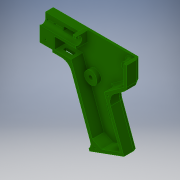
# Autodesk Inventor part: Griff_rechts
Saved by Autodesk Inventor 2019 (Build 230136000, 136)
## iProperties
Created: 2021-03-07
Part Number: Griff_rechts
Material: Generic
Document SubType Name: Modeling
Designer: Lukas
Density: 1 g/cm^3
Appearance: Default
Author: Lukas
Autodesk Inventor part; units mm, degrees
ref_plane "YZ Plane" through (0, 0, 0) normal (1, 0, 0) x (0, 1, 0)
ref_plane "XZ Plane" through (0, 0, 0) normal (0, 1, 0) x (-1, 0, 0)
ref_plane "XY Plane" through (0, 0, 0) normal (0, 0, 1) x (1, 0, 0)
sketch "Sketch1" plane through (0, 0, 0) normal (0, 0, 1) x (1, 0, 0)
  line L0 (-51.5891, 42.2862) -> (-20.8072, -42.2862)
  line L1 (-20.8072, -42.2862) -> (-24.5184, -46.7089)
  line L2 (-24.5184, -46.7089) -> (-23.4923, -49.528)
  line L3 (-23.4923, -49.528) -> (23.4923, -32.427)
  line L4 (27.261, 47.2862) -> (1.261, 28.653)
  line L5 (1.261, 28.653) -> (23.4923, -32.427)
  line L6 (0, -74.8908) -> (0, 102.649) projected
  line L7 (-91.5891, 77.2862) -> (27.261, 77.2862)
  line L8 (27.261, 77.2862) -> (27.261, 47.2862)
  line L9 (-51.5891, 42.2862) -> (-91.5891, 42.2862)
  line L10 (-91.5891, 42.2862) -> (-91.5891, 77.2862)
  point P0 (0, 0)
  point P1 (-36.1981, 0)
  point P2 (0, -40.9775)
  dimension "d1" = 90
  dimension "d2" = 120
  dimension "d3" = 3
  dimension "d5" = 45
  dimension "d6" = 20
  dimension "d7" = 65
  dimension "d8" = 5
  dimension "d10" = 30
  dimension "d30" = 26
  dimension "d31" = 40
  dimension "d32" = 35
  constraints: 21 end point, 5 perpendicular, 2 midpoint, 1 horizontal, 1 horizontal alignment, 1 parallel, 1 vertical alignment
  measures "d1" distance of L0.start L0.end
  measures "d2" angle of L0 L1
  measures "d3" distance of L1.end L2.end
  measures "d5" distance between parallel lines of L5 L0
  measures "d6" angle of L6 L0
  measures "d7" distance of L4.end L3.end
  measures "d8" distance between parallel lines of L2 L0
  measures "d10" distance of L7.end L4.start
  measures "d30" distance from line of L8 L4.end
  measures "d31" distance of L0.start L9.end
  measures "d32" distance of L9.end L7.start
extrude "Extrusion1" add sketch "Sketch1" along normal blind 2.5
sketch "Sketch2" plane through (0, 0, 2.5) normal (0, 0, 1) x (1, 0, 0)
  line L0 (-51.5891, 42.2862) -> (-20.8072, -42.2862) projected
  line L1 (-20.8072, -42.2862) -> (-24.5184, -46.7089) projected
  line L2 (-24.5184, -46.7089) -> (-23.4923, -49.528) projected
  line L3 (-23.4923, -49.528) -> (23.4923, -32.427) projected
  line L4 (23.4923, -32.427) -> (1.261, 28.653) projected
  line L5 (1.261, 28.653) -> (27.261, 47.2862) projected
  line L6 (27.261, 47.2862) -> (27.261, 77.2862) projected
  line L7 (27.261, 77.2862) -> (-91.5891, 77.2862) projected
  circle A0 centre (-32, 28) radius 3
  circle A1 centre (-32, 28) radius 8.5
  line L8 (-91.5891, 77.2862) -> (-91.5891, 42.2862) projected
  line L9 (-91.5891, 42.2862) -> (-51.5891, 42.2862) projected
  point P0 (0, 0)
  dimension "d55" = 6
  dimension "d56" = 17
  dimension "d126" = 28
  dimension "d127" = 32
  constraints: 2 centre point, 1 coincident
  measures "d55" diameter of A0
  measures "d56" diameter of A1
  measures "d126" vertical distance of point (0, 0) A0.centre
  measures "d127" horizontal distance of point (0, 0) A0.centre
extrude "Extrusion2" add sketch "Sketch2" along normal blind 6 contours A1
sketch "Sketch3" plane through (0, 0, 2.5) normal (0, 0, 1) x (1, 0, 0)
  line L0 (-51.5891, 42.2862) -> (-20.8072, -42.2862) projected
  line L1 (-20.8072, -42.2862) -> (-24.5184, -46.7089) projected
  line L2 (-24.5184, -46.7089) -> (-23.4923, -49.528) projected
  line L3 (-23.4923, -49.528) -> (23.4923, -32.427) projected
  line L4 (23.4923, -32.427) -> (1.261, 28.653) projected
  line L5 (1.261, 28.653) -> (27.261, 47.2862) projected
  line L6 (27.261, 47.2862) -> (27.261, 77.2862) projected
  line L7 (27.261, 77.2862) -> (-91.5891, 77.2862) projected
  circle A0 centre (-32, 28) radius 8.5 projected
  line L8 (-48.7882, 46.2862) -> (-16.4032, -42.6911)
  line L9 (-16.4032, -42.6911) -> (18.3655, -30.0363)
  line L10 (18.3655, -30.0363) -> (-3.5357, 30.1366)
  line L11 (-3.5357, 30.1366) -> (23.261, 49.3407)
  line L12 (23.261, 49.3407) -> (23.261, 77.2862)
  line L13 (27.261, 77.2862) -> (-91.5891, 77.2862) projected
  line L14 (1.261, 28.653) -> (27.261, 47.2862) projected
  line L15 (23.4923, -32.427) -> (1.261, 28.653) projected
  line L16 (-51.5891, 42.2862) -> (-20.8072, -42.2862) projected
  line L17 (-24.5184, -46.7089) -> (-20.8072, -42.2862) projected
  line L18 (-51.5891, 42.2862) -> (-20.8072, -42.2862)
  line L19 (-20.8072, -42.2862) -> (-24.5184, -46.7089)
  line L20 (-24.5184, -46.7089) -> (-23.4923, -49.528)
  line L21 (23.4923, -32.427) -> (-23.4923, -49.528)
  line L22 (-23.4923, -49.528) -> (23.4923, -32.427) projected
  line L23 (23.4923, -32.427) -> (1.261, 28.653)
  line L24 (1.261, 28.653) -> (27.261, 47.2862)
  line L25 (27.261, 77.2862) -> (27.261, 47.2862)
  line L26 (23.261, 77.2862) -> (27.261, 77.2862)
  line L27 (-91.5891, 77.2862) -> (-91.5891, 42.2862) projected
  line L28 (-91.5891, 42.2862) -> (-51.5891, 42.2862) projected
  line L29 (-91.5891, 77.2862) -> (-91.5891, 42.2862) projected
  line L30 (-51.5891, 42.2862) -> (-91.5891, 42.2862)
  line L31 (-91.5891, 42.2862) -> (-91.5891, 46.2862)
  line L32 (-91.5891, 46.2862) -> (-48.7882, 46.2862)
  point P0 (-51.5891, 77.2862)
  dimension "d20" = 4
  dimension "d21" = 4
  dimension "d22" = 4
  dimension "d23" = 4
  dimension "d24" = 4
  dimension "d33" = 4
  constraints: 32 end point, 6 perpendicular, 5 parallel, 2 point on line, 2 vertical, 1 collinear, 1 horizontal
  measures "d20" distance between parallel lines of L6 L12
  measures "d21" distance between parallel lines of L16 L8
  measures "d22" distance between parallel lines of L4 L10
  measures "d23" distance between parallel lines of L14 L11
  measures "d24" distance between parallel lines of L3 L9
  measures "d33" distance between parallel lines of L32 L28
extrude "Extrusion3" add sketch "Sketch3" along normal blind 16 contours L28 L27 L32 L8 L9 L10 L11 L12 L7 L6 L5 L4 L3 L2 L1 L0
fillet "Fillet3" radius 15 2 edges at (1.261, 28.653, 9.25) (-51.5891, 42.2862, 9.25)
fillet "Fillet1" radius 6 1 edges at (7.4149, 0.0501, 2.5)
fillet "Fillet2" radius 8 2 edges at (27.261, 47.2862, 9.25) (-20.8072, -42.2862, 9.25)
chamfer "Chamfer4" distance 10 angle 45 1 edges at (-16.4032, -42.6911, 10.5)
sketch "Sketch4" plane through (0, 0, 2.5) normal (0, 0, 1) x (1, 0, 0)
  line L0 (-91.5891, 77.2862) -> (-91.5891, 46.2862) projected
  line L1 (-91.5891, 77.2862) -> (-42.0891, 77.2862)
  line L2 (-42.0891, 77.2862) -> (-42.0891, 62.2862)
  line L3 (-42.0891, 62.2862) -> (-91.5891, 62.2862)
  line L4 (-91.5891, 62.2862) -> (-91.5891, 77.2862)
  line L5 (23.261, 77.2862) -> (-91.5891, 77.2862) projected
  line L6 (-48.7882, 46.2862) -> (-91.5891, 46.2862) projected
  point P0 (0, 0)
  point P1 (11.261, 77.2862)
  point P2 (-76.5891, 52.2862)
  point P3 (-59.2913, 46.2862)
  dimension "d34" = 49.5
  dimension "d42" = 16
  constraints: 8 end point, 2 parallel, 1 horizontal, 1 perpendicular, 1 other
  measures "d34" distance of L1.start L1.end
  measures "d42" distance between parallel lines of L6 L3
extrude "Extrusion4" add sketch "Sketch4" along normal blind 16
sketch "Sketch5" plane through (-91.5891, 77.2862, 0) normal (-1, 0, 0) x (0, 0, 1)
  circle A0 centre (15.5, -7.5) radius 5
  line L0 (18.5, 0) -> (18.5, -15) projected
  point P0 (0, -77.2862)
  point P1 (18.5, -7.5)
  dimension "d39" = 10
  dimension "d152" = 3
  constraints: 1 centre point, 1 horizontal alignment, 1 midpoint
  measures "d39" diameter of A0
  measures "d152" distance from line of L0 A0.centre
extrude "Extrusion5" cut sketch "Sketch5" against normal up to surface (49.5 mm away)
sketch "Sketch6" plane through (0, 0, 2.5) normal (0, 0, 1) x (1, 0, 0)
  line L0 (-42.0891, 62.2862) -> (-91.5891, 62.2862) projected
  line L1 (-91.5891, 62.2862) -> (-91.5891, 46.2862)
  line L2 (-71.5891, 46.2862) -> (-71.5891, 62.2862)
  line L3 (-91.5891, 62.2862) -> (-71.5891, 62.2862)
  line L4 (-71.5891, 46.2862) -> (-91.5891, 46.2862)
  point P0 (0, 0)
  dimension "d53" = 20
  constraints: 8 end point, 1 coincident, 1 collinear, 1 horizontal, 1 parallel, 1 perpendicular
  measures "d53" distance between parallel lines of L1 L2
extrude "Extrusion6" add sketch "Sketch6" along normal blind 16
sketch "Sketch10" plane through (0, 0, 18.5) normal (0, 0, 1) x (1, 0, 0)
  line L0 (-91.5891, 73.7862) -> (-42.0891, 73.7862) projected
  line L1 (-91.5891, 65.7862) -> (-91.5891, 73.7862) projected
  line L2 (-91.5891, 77.2862) -> (-91.5891, 73.7862) projected
  line L3 (-91.5891, 42.2862) -> (-91.5891, 77.2862) projected
  line L4 (-91.5891, 65.7862) -> (-91.5891, 42.2862) projected
  line L5 (-42.0891, 73.7862) -> (-42.0891, 65.7862) projected
  line L6 (-42.0891, 73.7862) -> (-42.0891, 77.2862) projected
  line L7 (-42.0891, 77.2862) -> (-42.0891, 62.2862) projected
  line L8 (-67.0891, 72.7862) -> (-47.0891, 72.7862)
  line L9 (-47.0891, 72.7862) -> (-47.0891, 66.7862)
  line L10 (-47.0891, 66.7862) -> (-67.0891, 66.7862)
  line L11 (-67.0891, 66.7862) -> (-67.0891, 72.7862)
  line L12 (-42.0891, 62.2862) -> (-42.0891, 65.7862) projected
  line L13 (-42.0891, 65.7862) -> (-91.5891, 65.7862) projected
  point P0 (0, 0)
  point P1 (-47.0891, 69.7862)
  point P2 (-42.0891, 69.7862)
  dimension "d67" = 1
  dimension "d69" = 6
  dimension "d70" = 5
  dimension "d71" = 20
  constraints: 8 end point, 2 midpoint, 2 parallel, 1 horizontal, 1 horizontal alignment, 1 perpendicular
  measures "d67" distance between parallel lines of L0 L8
  measures "d69" distance of L10.end L8.start
  measures "d70" distance between parallel lines of L5 L9
  measures "d71" distance of L8.start L8.end
extrude "Extrusion11" cut sketch "Sketch10" against normal through all contours L8 L9 L10 L11
sketch "Sketch11" plane through (0, 0, 2.5) normal (0, 0, 1) x (1, 0, 0)
  circle A0 centre (17.261, 67.2862) radius 5
  line L0 (23.261, 77.2862) -> (23.261, 49.3407) projected
  line L1 (23.261, 49.3407) -> (-3.5357, 30.1366) projected
  line L2 (10.5108, 35.282) -> (23.9211, 44.8926) projected
  arc A1 (23.9211, 44.8926) -> (27.261, 51.3952) centre (19.261, 51.3952) ccw projected
  line L3 (27.261, 51.3952) -> (27.261, 77.2862) projected
  line L4 (-91.5891, 77.2862) -> (27.261, 77.2862) projected
  line L5 (23.261, 77.2862) -> (-42.0891, 77.2862) projected
  line L6 (27.261, 77.2862) -> (23.261, 77.2862) projected
  line L7 (0.4724, 33.3853) -> (17.261, 49.0265) projected
  circle A2 centre (17.261, 67.2862) radius 1.45
  line L8 (27.261, 77.2862) -> (27.261, 51.3952) projected
  arc A3 (23.9211, 44.8926) -> (27.261, 51.3952) centre (19.261, 51.3952) ccw projected
  line L9 (23.9211, 44.8926) -> (10.5108, 35.282) projected
  line L10 (-8.5998, 26.5073) -> (23.261, 49.3407) projected
  line L11 (23.261, 49.3407) -> (23.261, 77.2862) projected
  line L12 (-42.0891, 77.2862) -> (-91.5891, 77.2862) projected
  line L13 (-3.5357, 30.1366) -> (-8.5998, 26.5073) projected
  point P0 (0, 0)
  dimension "d75" = 10
  dimension "d76" = 10
  dimension "d77" = 2.9
  dimension "d121" = 6
  constraints: 2 centre point, 1 coincident
  measures "d75" distance from line of L4 A0.centre
  measures "d76" diameter of A0
  measures "d77" diameter of A2
  measures "d121" distance from line of L0 A0.centre
extrude "Extrusion12" add sketch "Sketch11" along normal blind 8.5
sketch "Sketch17" plane through (0, 0, 2.5) normal (0, 0, 1) x (1, 0, 0)
  circle A0 centre (-59.5891, 58.2862) radius 4
  circle A1 centre (-59.5891, 58.2862) radius 1.45
  line L0 (-42.0891, 62.2862) -> (-71.5891, 62.2862) projected
  line L1 (-71.5891, 62.2862) -> (-42.0891, 62.2862) projected
  line L2 (-71.5891, 46.2862) -> (-71.5891, 62.2862) projected
  line L3 (-71.5891, 62.2862) -> (-71.5891, 46.2862) projected
  line L4 (-42.0891, 73.7862) -> (-42.0891, 65.7862) projected
  line L5 (-42.0891, 73.7862) -> (-42.0891, 77.2862) projected
  line L6 (-42.0891, 77.2862) -> (-42.0891, 62.2862) projected
  line L7 (-42.0891, 62.2862) -> (-42.0891, 65.7862) projected
  point P0 (0, 0)
  dimension "d109" = 2.9
  dimension "d110" = 8
  dimension "d111" = 4
  constraints: 2 centre point, 1 coincident
  measures "d109" diameter of A1
  measures "d110" diameter of A0
  measures "d111" distance from line of L0 A0.centre
extrude "Extrusion18" add sketch "Sketch17" along normal blind 3
sketch "Sketch12" plane through (23.261, 49.3407, 18.5) normal (-1, 0, 0) x (0, 0, 1)
  circle A0 centre (-4, 4) radius 3.5
  line L0 (0, 27.9455) -> (0, 0) projected
  line L1 (-16, 0) -> (0, 0) projected
  point P0 (-18.5, -49.3407)
  point P1 (-10, 0)
  dimension "d81" = 4
  dimension "d82" = 7
  dimension "d83" = 4
  constraints: 1 centre point
  measures "d81" distance from line of L0 A0.centre
  measures "d82" diameter of A0
  measures "d83" distance from line of L1 A0.centre
extrude "Extrusion13" cut sketch "Sketch12" against normal blind 2
sketch "Sketch14" plane through (-91.5891, 42.2862, 18.5) normal (0, -1, 0) x (1, 0, 0)
  line L0 (25, -6.3) -> (39, -6.3)
  line L1 (39, -6.3) -> (39, -11.5)
  line L2 (39, -11.5) -> (25, -11.5)
  line L3 (25, -11.5) -> (25, -6.3)
  line L4 (0, 0) -> (29.4969, 0) projected
  line L5 (0, -18.5) -> (0, 0) projected
  point P0 (91.5891, -18.5)
  point P1 (0, -12)
  dimension "d91" = 25
  dimension "d92" = 14
  dimension "d93" = 5.2
  dimension "d122" = 7
  constraints: 8 end point, 2 parallel, 1 perpendicular
  measures "d91" distance between parallel lines of L5 L3
  measures "d92" distance of L1.end L2.end
  measures "d93" distance of L0.end L1.end
  measures "d122" distance from line of L5.start L2
extrude "Extrusion15" cut sketch "Sketch14" against normal blind 4 and the other way blind 4
sketch "Sketch18" plane through (0, 0, 2.5) normal (0, 0, 1) x (1, 0, 0)
  line L0 (18.3655, -30.0363) -> (-3.5357, 30.1366) projected
  line L1 (-3.5357, 30.1366) -> (18.3655, -30.0363) projected
  line L2 (23.4923, -32.427) -> (5.1532, 17.9594) projected
  line L3 (5.1532, 17.9594) -> (23.4923, -32.427) projected
  line L4 (2.6207, 13.2221) -> (-8.6556, 9.1179)
  line L5 (-8.6556, 9.1179) -> (-3.5253, -4.9775)
  line L6 (-3.5253, -4.9775) -> (7.751, -0.8733)
  line L7 (7.751, -0.8733) -> (2.6207, 13.2221)
  point P0 (0, 0)
  dimension "d128" = 18
  dimension "d129" = 15
  dimension "d130" = 12
  constraints: 8 end point, 2 parallel, 2 point on line, 1 perpendicular
  measures "d128" distance from line of L0.end L4
  measures "d129" distance of L4.end L5.end
  measures "d130" distance of L5.end L6.end
extrude "Extrusion19" add sketch "Sketch18" along normal blind 8
fillet "Fillet4" radius 3 2 edges at (12.261, 67.2862, 2.5) (7.3306, 37.924, 2.5)
chamfer "Chamfer1" distance 1 distance2 4 1 edges at (-42.0891, 77.2862, 10.5) measured on face at (-42.0891, 76.7862, 10.5)
chamfer "Chamfer2" [suppressed]
chamfer "Chamfer3" distance 3 angle 60 10 edges at (-35.1919, -2.7647, 0) (-53.4885, 39.5734, 0) (-76.8406, 42.2862, 0) (-22.026, -42.0713, 0) (-24.1473, -46.2667, 0) (14.3227, -7.2338, 0) (4.9183, 27.5219, 0) (17.216, 40.0873, 0) (26.3772, 47.7401, 0) (27.261, 64.3407, 0) measured on face at (-76.8406, 42.7862, 0) measured on face at (4.4406, 27.6696, 0) measured on face at (-23.7642, -46.588, 0) measured on face at (-34.722, -2.5937, 0) measured on face at (-21.5336, -42.1581, 0) measured on face at (13.8529, -7.4048, 0) measured on face at (-53.2017, 39.983, 0) measured on face at (26.761, 64.3407, 0) measured on face at (25.9325, 47.9685, 0) measured on face at (16.9247, 40.4937, 0)
sketch "Sketch19" plane through (0, 0, 10.5) normal (0, 0, 1) x (1, 0, 0)
  circle A0 centre (0.3164, 4.9342) radius 1.9
  line L0 (-8.6556, 9.1179) -> (-3.5253, -4.9775) projected
  line L1 (2.6207, 13.2221) -> (-8.6556, 9.1179) projected
  point P0 (0, 0)
  dimension "d133" = 7
  dimension "d134" = 7
  dimension "d135" = 3.8
  constraints: 1 centre point
  measures "d133" distance from line of A0.centre L0
  measures "d134" distance from line of L1 A0.centre
  measures "d135" diameter of A0
extrude "Extrusion20" cut sketch "Sketch19" against normal blind 9.5
sketch "Sketch20" plane through (-91.5891, 77.2862, 0) normal (-1, 0, 0) x (0, 0, 1)
  line L0 (0, -32) -> (0, 0) projected
  line L1 (0, -29) -> (6, -29)
  line L2 (6, -29) -> (6, -19)
  line L3 (6, -19) -> (3, -19)
  line L4 (3, -19) -> (3, -4)
  line L5 (2.5, -11.45) -> (11, -11.45) projected
  line L6 (3, -4) -> (0, -4)
  line L7 (0, -4) -> (0, -29)
  line L8 (0, 0) -> (18.5, 0) projected
  line L9 (5.1962, -35) -> (18.5, -35) projected
  line L10 (11.5, -35) -> (19.5, -35)
  line L11 (19.5, -35) -> (19.5, -32)
  line L12 (19.5, -32) -> (11.5, -32)
  line L13 (11.5, -32) -> (11.5, -35)
  point P0 (0, -77.2862)
  dimension "d138" = 4
  dimension "d139" = 3
  dimension "d140" = 6
  dimension "d141" = 10
  dimension "d142" = 6
  dimension "d153" = 11.5
  dimension "d154" = 8
  dimension "d155" = 3
  constraints: 20 end point, 7 perpendicular, 2 parallel, 2 point on line, 1 horizontal
  measures "d138" distance between parallel lines of L8 L6
  measures "d139" distance of L4.end L6.end
  measures "d140" distance between parallel lines of L9 L1
  measures "d141" distance of L1.end L2.end
  measures "d142" distance of L1.start L1.end
  measures "d153" distance between parallel lines of L7 L13
  measures "d154" distance of L11.end L12.end
  measures "d155" distance of L12.end L10.start
extrude "Extrusion21" cut sketch "Sketch20" against normal blind 17.25
sketch "Sketch22" plane through (-91.5891, 45.2862, 11.5) normal (0, -1, 0) x (1, 0, 0)
  circle A0 centre (4, 4) radius 1.35
  circle A1 centre (12, 4) radius 1.35
  line L0 (0, 0) -> (0, 7) projected
  point P0 (91.5891, -11.5)
  point P1 (0, -11.5)
  dimension "d156" = 4
  dimension "d157" = 2.7
  dimension "d158" = 8
  dimension "d159" = 15.5
  constraints: 2 centre point, 1 equal radius, 1 horizontal alignment
  measures "d156" distance from line of L0 A0.centre
  measures "d157" diameter of A0
  measures "d158" distance of A1.centre A0.centre
  measures "d159" vertical distance of point (0, -11.5) A0.centre
extrude "Extrusion23" cut sketch "Sketch22" against normal blind 15
sketch "Sketch21" plane through (-91.5891, 58.2862, 3) normal (0, 0, -1) x (-1, 0, 0)
  circle A0 centre (-13, 11) radius 1.35
  circle A1 centre (-3, 11) radius 1.35
  circle A2 centre (-3, 4) radius 1.35
  circle A3 centre (-13, 4) radius 1.35
  line L0 (0, 0) -> (-17.25, 0) projected
  line L1 (0, 15) -> (-17.25, 15) projected
  line L2 (0, 15) -> (0, 0) projected
  point P0 (-91.5891, -58.2862)
  dimension "d145" = 2.7
  dimension "d146" = 4
  dimension "d147" = 4
  dimension "d148" = 3
  dimension "d149" = 10
  constraints: 4 centre point, 3 equal radius, 2 horizontal alignment, 2 vertical alignment
  measures "d145" diameter of A1
  measures "d146" distance from line of L0 A2.centre
  measures "d147" distance from line of L1 A1.centre
  measures "d148" distance from line of L2 A1.centre
  measures "d149" distance of A1.centre A0.centre
extrude "Extrusion22" cut sketch "Sketch21" against normal blind 9
sketch "Sketch23" plane through (23.261, 77.2862, 18.5) normal (0, 1, 0) x (1, 0, 0)
  line L0 (-114.8501, 18.5) -> (-114.8501, 0) projected
  line L1 (-69.3501, 0) -> (-114.8501, 0) projected
  line L2 (-114.8501, 8) -> (-69.3501, 8)
  line L3 (-69.3501, 8) -> (-69.3501, 0)
  line L4 (-69.3501, 0) -> (-114.8501, 0)
  line L5 (-114.8501, 0) -> (-114.8501, 8)
  point P0 (-23.261, 18.5)
  dimension "d162" = 8
  dimension "d163" = 45.5
  constraints: 8 end point, 2 parallel, 2 point on line, 1 horizontal, 1 perpendicular
  measures "d162" distance between parallel lines of L1 L2
  measures "d163" distance of L2.start L2.end
extrude "Extrusion24" cut sketch "Sketch23" against normal blind 7.5
sketch "Sketch24" plane through (0, 0, 18.5) normal (0, 0, 1) x (1, 0, 0)
  circle A0 centre (1, 28) radius 1.35
  circle A1 centre (-16, -42) radius 1.35
  circle A2 centre (-83.5891, 52.2862) radius 1.35
  line L0 (-91.5891, 65.7862) -> (-91.5891, 45.2862) projected
  line L1 (-74.3391, 42.2862) -> (-62.0922, 42.2862) projected
  point P0 (0, 0)
  dimension "d166" = 2.7
  dimension "d167" = 28
  dimension "d168" = 1
  dimension "d171" = 42
  dimension "d172" = 16
  dimension "d180" = 8
  dimension "d181" = 10
  constraints: 3 centre point, 2 equal radius
  measures "d166" diameter of A0
  measures "d167" vertical distance of A0.centre point (0, 0)
  measures "d168" horizontal distance of point (0, 0) A0.centre
  measures "d171" vertical distance of point (0, 0) A1.centre
  measures "d172" horizontal distance of point (0, 0) A1.centre
  measures "d180" distance from line of L0 A2.centre
  measures "d181" distance from line of L1 A2.centre
extrude "Extrusion25" cut sketch "Sketch24" against normal blind 15
equation "\"d21\" = d20"
equation "\"d22\" = d20"
equation "\"d23\" = d20"
equation "\"d24\" = d20"
equation "\"d33\" = d20"
body "Solid1"
